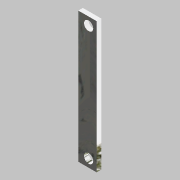
# Autodesk Inventor part: Tritt
Saved by Autodesk Inventor 2015 (Build 190159000, 159)
## iProperties
Created: 2017-04-11
Part Number: Tritt
Material: Generic
Document SubType Name: Modeling
Designer: Seelenernter
Density: 1 g/cm^3
Appearance: Chrom - poliert
Author: Seelenernter
Autodesk Inventor part; units mm, degrees
ref_plane "YZ Plane" through (0, 0, 0) normal (1, 0, 0) x (0, 1, 0)
ref_plane "XZ Plane" through (0, 0, 0) normal (0, 1, 0) x (-1, 0, 0)
ref_plane "XY Plane" through (0, 0, 0) normal (0, 0, 1) x (1, 0, 0)
sketch "Skizze1" plane through (0, 0, 0) normal (0, 1, 0) x (-1, 0, 0)
  line L0 (-40, 285) -> (40, 285)
  line L1 (40, 285) -> (40, -285)
  line L2 (40, -285) -> (-40, -285)
  line L3 (-40, -285) -> (-40, 285)
  line L4 (-40, 285) -> (40, -285) construction
  line L5 (40, 285) -> (-40, -285) construction
  point P0 (0, 0)
  dimension "d0" = 80
  dimension "d1" = 570
  constraints: 12 end point, 2 midpoint, 2 parallel, 1 horizontal, 1 perpendicular
  measures "d0" distance of L1.end L2.end
  measures "d1" distance of L0.end L1.end
extrude "Extrusion1" add sketch "Skizze1" along normal blind 20
sketch "Skizze2" plane through (0, 20, 0) normal (0, 1, 0) x (1, 0, 0)
  line L0 (-40, -285) -> (40, -285) projected
  line L1 (40, -285) -> (40, 285) projected
  line L2 (40, 285) -> (-40, 285) projected
  line L3 (-40, 285) -> (-40, -285) projected
  circle A0 centre (5, -250) radius 20
  point P0 (0, 0)
  dimension "d4" = 35
  dimension "d5" = 35
  dimension "d6" = 40
  constraints: 1 centre point
  measures "d4" distance from line of L1 A0.centre
  measures "d5" distance from line of L0 A0.centre
  measures "d6" diameter of A0
extrude "Extrusion2" cut sketch "Skizze2" against normal blind 20 contours A0
mirror "Spiegeln1" about plane through (0, 0, 0) normal (0, 0, 1) of "Extrusion2"
sketch "Skizze3" plane through (0, 20, 0) normal (0, 1, 0) x (1, 0, 0)
  circle A0 centre (-25, -195) radius 5
  line L0 (-40, -285) -> (40, -285) projected
  line L1 (-40, 285) -> (-40, -285) projected
  circle A1 centre (25, -195) radius 5
  line L2 (40, -285) -> (40, 285) projected
  circle A2 centre (0, -165) radius 5
  circle A3 centre (0, -110) radius 5
  circle A4 centre (0, -55) radius 5
  circle A5 centre (0, 0) radius 5
  circle A6 centre (0, 55) radius 5
  circle A7 centre (0, 110) radius 5
  circle A8 centre (0, 165) radius 5
  circle A9 centre (-25, -140) radius 5
  circle A10 centre (25, -140) radius 5
  circle A11 centre (-25, -85) radius 5
  circle A12 centre (25, -85) radius 5
  circle A13 centre (-25, -30) radius 5
  circle A14 centre (25, -30) radius 5
  circle A15 centre (-25, 25) radius 5
  circle A16 centre (25, 25) radius 5
  circle A17 centre (-25, 80) radius 5
  circle A18 centre (25, 80) radius 5
  circle A19 centre (-25, 135) radius 5
  circle A20 centre (25, 135) radius 5
  circle A21 centre (-25, 190) radius 5
  circle A22 centre (25, 190) radius 5
  point P0 (0, 0)
  dimension "d9" = 10
  dimension "d10" = 90
  dimension "d11" = 15
  dimension "d12" = 10
  dimension "d13" = 90
  dimension "d14" = 15
  dimension "d15" = 10
  dimension "d16" = 120
  dimension "d19" = 55
  dimension "d26" = 55
  constraints: 23 centre point, 2 vertical, 40 other
  measures "d9" diameter of A0
  measures "d10" distance from line of L0 A0.centre
  measures "d11" distance from line of A0.centre L1
  measures "d12" diameter of A1
  measures "d13" distance from line of L0 A1.centre
  measures "d14" distance from line of L2 A1.centre
  measures "d15" diameter of A2
  measures "d16" distance from line of L0 A2.centre
  measures "d19" distance of A2.centre A3.centre
  measures "d26" distance of A0.centre A9.centre
extrude "Extrusion3" add sketch "Skizze3" along normal blind 2
fillet "Rundung1" radius 2 46 edges at (-30, 22, 195) (-30, 22, 140) (-5, 22, 165) (20, 22, 195) (20, 22, 140) (-5, 22, 110) (-30, 22, 85) (20, 22, 85) (-5, 22, 55) (-30, 22, 30) (20, 22, 30) (-5, 22, 0) (-30, 22, -25) (20, 22, -25) (-5, 22, -55) (-30, 22, -80) (20, 22, -80) (-5, 22, -110) (-30, 22, -135) (20, 22, -135) (-5, 22, -165) (-30, 22, -190) (20, 22, -190) (20, 20, -190) (-5, 20, -165) (-30, 20, -190) (-30, 20, -135) (-5, 20, -110) (20, 20, -135) (-30, 20, -80) (-5, 20, -55) (20, 20, -80) (20, 20, -25) (-5, 20, 0) (-30, 20, -25) (-30, 20, 30) (20, 20, 30) (-5, 20, 55) (-30, 20, 85) (-5, 20, 110) (20, 20, 85) (20, 20, 140) (-5, 20, 165) (-30, 20, 140) (-30, 20, 195) (20, 20, 195)
sketch "Skizze4" plane through (0, 20, 0) normal (0, 1, 0) x (1, 0, 0)
  line L0 (40, -285) -> (-40, -285) projected
  line L1 (-37, -285) -> (-37, 285)
  line L2 (-40, 285) -> (40, 285) projected
  line L3 (-35, 285) -> (-35, -285)
  point P0 (0, 0)
  dimension "d34" = 3
  dimension "d35" = 2
  constraints: 4 end point, 4 point on line, 1 parallel, 1 vertical
  measures "d34" distance from line of L0.end L1
  measures "d35" distance between parallel lines of L1 L3
extrude "Extrusion4" cut sketch "Skizze4" against normal blind 1
sketch "Skizze5" plane through (-40, 0, 285) normal (0, 0, 1) x (1, 0, 0)
  line L0 (3, 19) -> (3, 20) projected
  line L1 (0, 20) -> (3, 20) projected
  line L2 (0, 0) -> (0, 20) projected
  line L3 (80, 0) -> (0, 0) projected
  line L4 (80, 0) -> (80, 20) projected
  line L5 (5, 20) -> (80, 20) projected
  line L6 (5, 20) -> (5, 19) projected
  line L7 (5, 19) -> (3, 19) projected
  line L8 (3, 19) -> (3, 0)
  line L9 (0, 0) -> (80, 0) projected
  line L10 (5, 19) -> (5, 0)
  point P0 (40, 0)
  constraints: 4 end point, 2 point on line, 1 parallel, 1 vertical
extrude "Extrusion5" cut sketch "Skizze5" against normal blind 1 contours L7 L10 L3 L8
sketch "Skizze6" plane through (40, 0, -285) normal (0, 0, -1) x (-1, 0, 0)
  line L0 (77, 20) -> (77, 19) projected
  line L1 (77, 19) -> (75, 19) projected
  line L2 (75, 19) -> (75, 20) projected
  line L3 (0, 20) -> (75, 20) projected
  line L4 (0, 0) -> (0, 20) projected
  line L5 (80, 0) -> (0, 0) projected
  line L6 (80, 0) -> (80, 20) projected
  line L7 (77, 20) -> (80, 20) projected
  line L8 (75, 19) -> (75, 0)
  line L9 (77, 19) -> (77, 0)
  line L10 (80, 0) -> (0, 0) projected
  point P0 (40, 0)
  constraints: 4 end point, 1 perpendicular, 1 point on line, 1 vertical
extrude "Extrusion6" cut sketch "Skizze6" against normal blind 1 contours L9 L5 L8 L1
